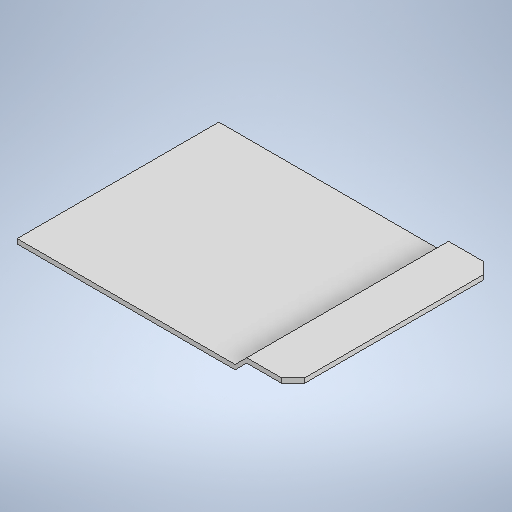
# Autodesk Inventor part: Part2
Saved by Autodesk Inventor 2025.2 (Build 292293000, 293)
## iProperties
Created: 2025-06-05
Part Number: Part2
Material: Generic
Document SubType Name: Sheet Metal
Designer: ziyuz
Density: 1 g/cm^3
Sheet Metal Rule: Default_mm
Appearance: Default
Author: ziyuz
Autodesk Inventor part; units mm, degrees
ref_plane "YZ Plane" through (0, 0, 0) normal (1, 0, 0) x (0, 1, 0)
ref_plane "XZ Plane" through (0, 0, 0) normal (0, 1, 0) x (-1, 0, 0)
ref_plane "XY Plane" through (0, 0, 0) normal (0, 0, 1) x (1, 0, 0)
sketch "Sketch1" plane through (0, 0, 0) normal (0, 1, 0) x (-1, 0, 0)
  line L0 (0, 0) -> (-94, 0)
  line L1 (-94, 0) -> (-94, -87)
  line L2 (-94, -87) -> (0, -87)
  line L3 (0, -87) -> (0, 0)
  dimension "d0" = 94
  dimension "d1" = 87
  constraints: 8 end point, 2 parallel, 1 horizontal, 1 perpendicular
  measures "d0" distance of L2.end L1.end
  measures "d1" distance of L1.end L0.end
extrude "Extrusion1" add sketch "Sketch1" along normal blind 2
sketch "Sketch2" plane through (0, 0, 0) normal (0, 0, 1) x (1, 0, 0)
  line L0 (94, 2) -> (0, 2) projected
  line L1 (-0.0001, 2) -> (94, 2)
  line L2 (94, 2) -> (99, 7)
  line L3 (94, 2) -> (101.071, 2) construction
  line L4 (94, 0) -> (99, 5)
  line L5 (99, 5) -> (114, 5)
  line L6 (114, 5) -> (114, 7)
  line L7 (114, 7) -> (99, 7)
  line L8 (94, 0) -> (94, 2) projected
  line L9 (94, 0) -> (94, 2)
  point P0 (0, 0)
  dimension "d4" = 7.071
  dimension "d5" = 45
  dimension "d6" = 7.071
  dimension "d7" = 15
  dimension "d8" = 2
  constraints: 16 end point, 3 horizontal, 2 perpendicular, 1 collinear, 1 equal length
  measures "d4" distance of L0.start L2.end
  measures "d5" angle of L3 L2
  measures "d6" distance of L4.start L4.end
  measures "d7" distance of L4.end L5.end
  measures "d8" distance of L5.end L6.end
extrude "Extrusion2" add sketch "Sketch2" against normal blind 87
sketch "Sketch3" plane through (99, 7, 0) normal (0, 1, 0) x (1, 0, 0)
  line L0 (15, 0) -> (0, 0) projected
  line L1 (15, 0) -> (20, 5)
  line L2 (15, 0) -> (22.071, 0) construction
  line L3 (20, 5) -> (20, 82)
  line L4 (0, 87) -> (15, 87) projected
  line L5 (20, 82) -> (15, 87)
  line L6 (15, 0) -> (15, 87)
  point P0 (-99, 0)
  dimension "d11" = 7.071
  dimension "d12" = 45
  dimension "d13" = 77
  constraints: 10 end point, 1 equal length, 1 horizontal, 1 vertical
  measures "d11" distance of L0.start L1.end
  measures "d12" angle of L2 L1
  measures "d13" distance of L1.end L3.end
extrude "Extrusion3" add sketch "Sketch3" against normal blind 2
equation "\"BendRadius\" = Thickness"
equation "\"BendReliefWidth\" = Thickness"
equation "\"BendReliefDepth\" = 0.5 * Thickness"
equation "\"CornerReliefSize\" = 4 * Thickness"
equation "\"MinimumRemnant\" = 2 * Thickness"
equation "\"TransitionRadius\" = BendRadius"
equation "\"JacobiRadiusSize\" = BendRadius"
equation "\"GapSize\" = Thickness"
equation "\"Thickness\" = 0.5"
body "Solid1"
